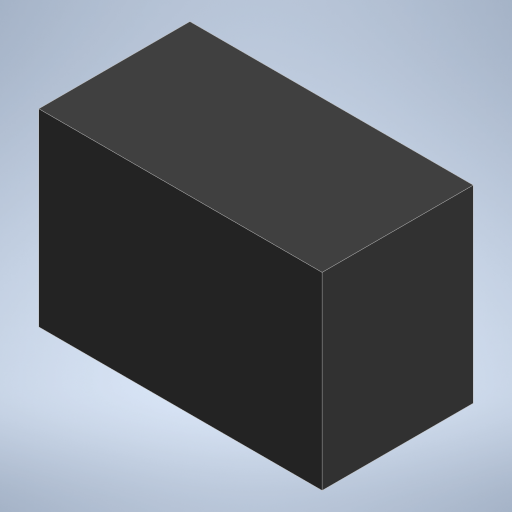
# Autodesk Inventor part: nitrile_rubber
Saved by Autodesk Inventor 2024 (Build 280153000, 153)
## iProperties
Created: 2025-05-23
Part Number: nitrile_rubber
Material: ゴム、ニトリル
Document SubType Name: Modeling
Designer: 1412z
Density: 1.2 g/cm^3
Appearance: ゴム - 黒
Author: 1412z
Autodesk Inventor part; units mm, degrees
ref_plane "YZ Plane" through (0, 0, 0) normal (1, 0, 0) x (0, 1, 0)
ref_plane "XZ Plane" through (0, 0, 0) normal (0, 1, 0) x (-1, 0, 0)
ref_plane "XY Plane" through (0, 0, 0) normal (0, 0, 1) x (1, 0, 0)
sketch "スケッチ1" plane through (0, 0, 0) normal (0, 0, 1) x (1, 0, 0)
  line L0 (-7.5, 5) -> (7.5, 5)
  line L1 (7.5, 5) -> (7.5, -5)
  line L2 (7.5, -5) -> (-7.5, -5)
  line L3 (-7.5, -5) -> (-7.5, 5)
  line L4 (-7.5, 5) -> (7.5, -5) construction
  line L5 (7.5, 5) -> (-7.5, -5) construction
  point P0 (0, 0)
  dimension "d0" = 15
  dimension "d1" = 10
  constraints: 12 end point, 2 midpoint, 2 parallel, 1 horizontal, 1 perpendicular
  measures "d0" distance of L1.end L2.end
  measures "d1" distance of L0.end L1.end
extrude "押し出し1" add sketch "スケッチ1" along normal blind 8
